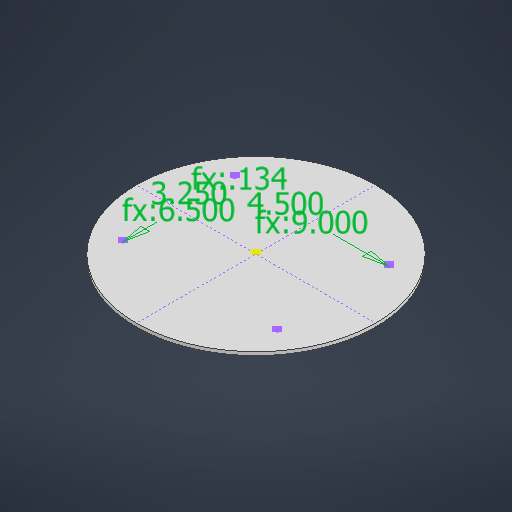
# Autodesk Inventor part: layer3_new
Saved by Autodesk Inventor 2026 (Build 300175050, 175E)
## iProperties
Created: 2025-06-05
Part Number: layer3_new
Material: Generic
Document SubType Name: Modeling
Designer: satom
Density: 1 g/cm^3
Appearance: Default
Author: satom
Autodesk Inventor part; units mm, degrees
ref_plane "YZ Plane" through (0, 0, 0) normal (1, 0, 0) x (0, 1, 0)
ref_plane "XZ Plane" through (0, 0, 0) normal (0, 1, 0) x (-1, 0, 0)
ref_plane "XY Plane" through (0, 0, 0) normal (0, 0, 1) x (1, 0, 0)
sketch "Sketch1" plane through (0, 0, 0) normal (0, 1, 0) x (-1, 0, 0)
  circle A0 centre (0, 0) radius 177
  dimension "d0" = 354
  constraints: 1 centre point, 1 coincident
  measures "d0" diameter of A0
extrude "Extrusion1" add sketch "Sketch1" along normal blind 5
sketch "Sketch2" plane through (0, 5, 0) normal (0, 1, 0) x (1, 0, 0)
  circle A0 centre (-114.3, 82.55) radius 1.7
  line L0 (-177, 0) -> (177, 0) construction
  line L1 (0, 177) -> (0, -177) construction
  circle A1 centre (114.3, 82.55) radius 1.7
  circle A2 centre (-114.3, -82.55) radius 1.7
  circle A3 centre (114.3, -82.55) radius 1.7
  point P0 (0, 0)
  dimension "d3" = 3.4
  dimension "d20" = 82.55
  dimension "d21" = 114.3
  dimension "d24" = 228.6
  dimension "d27" = 165.1
  constraints: 4 centre point, 4 end point, 2 horizontal, 2 vertical, 6 other
  measures "d3" diameter of A0
  measures "d20" distance from line of L0 A0.centre
  measures "d21" distance from line of L1 A0.centre
  measures "d24" distance of A0.centre A1.centre
  measures "d27" distance of A0.centre A2.centre
equation "\"d0\" = robot_diameter"
equation "\"d1\" = hardboard_thickness"
equation "\"d3\" = m3_clearance"
equation "\"d24\" = 2 * d21"
equation "\"d27\" = 2 * d20"
equation "\"m3_heat_set_insert\" = 4"
equation "\"m3_clearance\" = 3.4"
equation "\"m3_heat_set_depth\" = 7"
equation "\"robot_diameter\" = 354"
equation "\"hardboard_thickness\" = 5"
body "Solid1"
